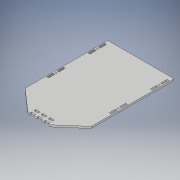
# Autodesk Inventor part: base
Saved by Autodesk Inventor 2018 (Build 220112000, 112)
## iProperties
Created: 2018-03-27
Part Number: base
Material: Generic
Document SubType Name: Modeling
Designer: guita
Density: 1 g/cm^3
Appearance: Default
Author: guita
Autodesk Inventor part; units mm, degrees
ref_plane "YZ Plane" through (0, 0, 0) normal (1, 0, 0) x (0, 1, 0)
ref_plane "XZ Plane" through (0, 0, 0) normal (0, 1, 0) x (-1, 0, 0)
ref_plane "XY Plane" through (0, 0, 0) normal (0, 0, 1) x (1, 0, 0)
sketch "Sketch1" plane through (0, 0, 0) normal (0, 1, 0) x (-1, 0, 0)
  point P0 (0, 0)
sketch "Sketch4" plane through (0, 0, 0) normal (0, 1, 0) x (-1, 0, 0)
  line L0 (-203.2, 0) -> (-203.2, -254)
  line L1 (-203.2, -254) -> (0, -254)
  line L2 (0, -254) -> (0, 0)
  line L3 (-101.6, 44.45) -> (-50.8, 44.45)
  line L4 (-50.8, 44.45) -> (0, 0)
  line L5 (-101.6, 44.45) -> (-152.4, 44.45)
  line L6 (-152.4, 44.45) -> (-203.2, 0)
  line L7 (-152.4, 44.45) -> (-136.0714, 58.7375)
  line L8 (-50.8, 44.45) -> (-67.1286, 58.7375)
  line L9 (-67.1286, 58.7375) -> (-136.0714, 58.7375)
  line L10 (0, -254) -> (0, -241.3)
  line L11 (-3.175, -241.3) -> (-3.175, -222.25)
  line L12 (-3.175, -222.25) -> (-9.525, -222.25)
  line L13 (-9.525, -222.25) -> (-9.525, -241.3)
  line L14 (-9.525, -241.3) -> (-3.175, -241.3)
  circle A0 centre (-6.35, -215.9) radius 4.7625
  circle A1 centre (-6.35, -215.9) radius 1.9844
  line L15 (-6.35, -209.55) -> (-9.525, -209.55)
  line L16 (-6.35, -209.55) -> (-3.175, -209.55)
  line L17 (-3.175, -209.55) -> (-3.175, -190.5)
  line L18 (-3.175, -190.5) -> (-9.525, -190.5)
  line L19 (-9.525, -190.5) -> (-9.525, -209.55)
  line L20 (-200.025, -241.3) -> (-200.025, -222.25)
  line L21 (-200.025, -222.25) -> (-193.675, -222.25)
  line L22 (-193.675, -222.25) -> (-193.675, -241.3)
  line L23 (-193.675, -241.3) -> (-200.025, -241.3)
  circle A2 centre (-196.85, -215.9) radius 4.7625
  circle A3 centre (-196.85, -215.9) radius 1.9844
  line L24 (-196.85, -209.55) -> (-193.675, -209.55)
  line L25 (-196.85, -209.55) -> (-200.025, -209.55)
  line L26 (-200.025, -209.55) -> (-200.025, -190.5)
  line L27 (-200.025, -190.5) -> (-193.675, -190.5)
  line L28 (-193.675, -190.5) -> (-193.675, -209.55)
  line L29 (-3.175, -63.5) -> (-3.175, -82.55)
  line L30 (-3.175, -82.55) -> (-9.525, -82.55)
  line L31 (-9.525, -82.55) -> (-9.525, -63.5)
  line L32 (-9.525, -63.5) -> (-3.175, -63.5)
  circle A4 centre (-6.35, -88.9) radius 4.7625
  circle A5 centre (-6.35, -88.9) radius 1.9844
  line L33 (-6.35, -95.25) -> (-9.525, -95.25)
  line L34 (-6.35, -95.25) -> (-3.175, -95.25)
  line L35 (-3.175, -95.25) -> (-3.175, -114.3)
  line L36 (-3.175, -114.3) -> (-9.525, -114.3)
  line L37 (-9.525, -114.3) -> (-9.525, -95.25)
  line L38 (-193.675, -63.5) -> (-200.025, -63.5)
  line L39 (-200.025, -63.5) -> (-200.025, -82.55)
  line L40 (-193.675, -82.55) -> (-193.675, -63.5)
  line L41 (-200.025, -82.55) -> (-193.675, -82.55)
  circle A6 centre (-196.85, -88.9) radius 4.7625
  line L42 (-196.85, -95.25) -> (-200.025, -95.25)
  line L43 (-196.85, -95.25) -> (-193.675, -95.25)
  line L44 (-200.025, -95.25) -> (-200.025, -114.3)
  line L45 (-200.025, -114.3) -> (-193.675, -114.3)
  line L46 (-193.675, -114.3) -> (-193.675, -95.25)
  circle A7 centre (-196.85, -88.9) radius 1.9844
  dimension "d18" = 203.2
  dimension "d19" = 254
  dimension "d29" = 19.05
  dimension "d30" = 6.35
  dimension "d32" = 9.525
  dimension "d33" = 3.9688
  dimension "d35" = 3.175
  dimension "d36" = 19.05
  constraints: 94 end point, 8 centre point, 6 perpendicular, 5 horizontal, 4 coincident, 2 parallel, 2 point on line
  measures "d18" distance of L1.end L0.end
  measures "d19" distance of L0.end L0.start
  measures "d29" distance of L11.start L11.end
  measures "d30" distance of L11.end L12.end
  measures "d32" diameter of A0
  measures "d33" diameter of A1
  measures "d35" distance of L15.start L16.end
  measures "d36" distance of L16.end L17.end
extrude "Extrusion2" add sketch "Sketch4" along normal blind 5.5563 contours L6 L5 L3 L4 L2 L1 L0 | L7 L9 L8 L3 L5 | A0 | A2 | A4 | A6
sketch "Sketch5" plane through (0, 5.5563, 0) normal (0, 1, 0) x (1, 0, 0)
  line L0 (67.1286, -58.7375) -> (136.0714, -58.7375) projected
  line L1 (136.0714, -58.7375) -> (129.7214, -58.7375)
  line L2 (129.7214, -58.7375) -> (129.7214, -52.3875)
  line L3 (129.7214, -52.3875) -> (117.0214, -52.3875)
  line L4 (117.0214, -52.3875) -> (117.0214, -58.7375)
  line L5 (117.0214, -58.7375) -> (104.3214, -58.7375)
  line L6 (0, 0) -> (67.1286, -58.7375) projected
  line L7 (67.1286, -58.7375) -> (73.4786, -58.7375)
  line L8 (73.4786, -58.7375) -> (73.4786, -52.3875)
  line L9 (73.4786, -52.3875) -> (86.1786, -52.3875)
  line L10 (86.1786, -52.3875) -> (86.1786, -58.7375)
  line L11 (86.1786, -58.7375) -> (101.5964, -58.7375)
  line L12 (101.5964, -52.3875) -> (95.2464, -52.3875)
  line L13 (101.5964, -52.3875) -> (107.9464, -52.3875)
  line L14 (107.9464, -52.3875) -> (107.9464, -58.7375)
  line L15 (95.2464, -52.3875) -> (95.2464, -58.7375)
  line L16 (73.4786, -58.7375) -> (86.1786, -58.7375)
  constraints: 30 end point, 8 perpendicular, 7 point on line, 1 collinear, 1 horizontal
extrude "Extrusion3" cut sketch "Sketch5" against normal blind 25.4
sketch "Sketch6" plane through (0, 5.5563, 0) normal (0, 1, 0) x (1, 0, 0)
  line L0 (73.4786, -52.3875) -> (86.1786, -52.3875) projected
  line L1 (73.4786, -46.0375) -> (73.4786, -39.6875)
  line L2 (73.4786, -39.6875) -> (73.4786, -46.0375)
  line L3 (129.74, -46.0375) -> (129.74, -39.6875)
  line L4 (129.74, -39.6875) -> (129.74, -46.0375)
  line L5 (86.1786, -46.0375) -> (86.1786, -39.6875)
  line L6 (95.2464, -46.0375) -> (95.2464, -39.6875)
  line L7 (117.0167, -46.0375) -> (117.0167, -39.6875)
  line L8 (107.95, -46.0375) -> (107.95, -39.6875)
  line L9 (73.4786, -39.6875) -> (86.1786, -39.6875)
  line L10 (95.2464, -39.6875) -> (107.95, -39.6875)
  line L11 (117.0167, -39.6875) -> (129.74, -39.6875)
  line L12 (129.74, -46.0375) -> (117.0167, -46.0375)
  line L13 (107.95, -46.0375) -> (95.2464, -46.0375)
  line L14 (86.1786, -46.0375) -> (73.4786, -46.0375)
  point P0 (0, 0)
  point P1 (95.2464, -52.3875)
  constraints: 28 end point, 15 perpendicular, 2 vertical
extrude "Extrusion4" cut sketch "Sketch6" against normal blind 25.4
sketch "Sketch7" plane through (0, 5.5563, 0) normal (0, 1, 0) x (1, 0, 0)
  line L0 (3.175, 63.5) -> (3.175, 82.55) projected
  line L1 (3.175, 73.025) -> (8.7313, 73.025)
  line L2 (9.525, 82.55) -> (3.175, 82.55) projected
  line L3 (3.175, 63.5) -> (9.525, 63.5) projected
  line L4 (9.525, 82.55) -> (8.7313, 82.55)
  line L5 (8.7313, 82.55) -> (8.7313, 63.5)
  line L6 (8.7313, 63.5) -> (9.525, 63.5)
  line L7 (9.525, 63.5) -> (9.525, 82.55)
  line L8 (9.525, 114.3) -> (8.7313, 114.3)
  line L9 (8.7313, 114.3) -> (8.7313, 95.25)
  line L10 (8.7313, 95.25) -> (9.525, 95.25)
  line L11 (9.525, 95.25) -> (9.525, 114.3)
  line L12 (3.175, 209.55) -> (9.525, 209.55) projected
  line L13 (3.175, 190.5) -> (9.525, 190.5) projected
  line L14 (9.525, 209.55) -> (8.7313, 209.55)
  line L15 (8.7313, 209.55) -> (8.7313, 190.5)
  line L16 (8.7313, 190.5) -> (9.525, 190.5)
  line L17 (9.525, 190.5) -> (9.525, 209.55)
  line L18 (9.525, 241.3) -> (9.525, 222.25) projected
  line L19 (9.525, 241.3) -> (9.1281, 241.3)
  line L20 (9.1281, 222.25) -> (9.525, 222.25)
  line L21 (9.525, 222.25) -> (9.525, 241.3)
  line L22 (3.175, 222.25) -> (3.175, 241.3) projected
  line L23 (9.525, 241.3) -> (8.7313, 241.3)
  line L24 (8.7313, 241.3) -> (8.7313, 222.25)
  line L25 (8.7313, 222.25) -> (9.525, 222.25)
  line L26 (9.525, 222.25) -> (9.525, 241.3)
  line L27 (200.025, 241.3) -> (200.025, 222.25) projected
  line L28 (200.025, 231.775) -> (194.4688, 231.775)
  line L29 (193.675, 241.3) -> (193.675, 222.25) projected
  line L30 (193.675, 241.3) -> (194.4688, 241.3)
  line L31 (194.4688, 241.3) -> (194.4688, 222.25)
  line L32 (194.4688, 222.25) -> (193.675, 222.25)
  line L33 (193.675, 222.25) -> (193.675, 241.3)
  line L34 (193.675, 209.55) -> (193.675, 190.5) projected
  line L35 (200.025, 190.5) -> (193.675, 190.5) projected
  line L36 (193.675, 209.55) -> (194.4688, 209.55)
  line L37 (194.4688, 209.55) -> (194.4688, 190.5)
  line L38 (194.4688, 190.5) -> (193.675, 190.5)
  line L39 (193.675, 190.5) -> (193.675, 209.55)
  line L40 (193.675, 114.3) -> (194.4688, 114.3)
  line L41 (194.4688, 114.3) -> (194.4688, 95.25)
  line L42 (194.4688, 95.25) -> (193.675, 95.25)
  line L43 (193.675, 95.25) -> (193.675, 114.3)
  line L44 (193.675, 82.55) -> (193.675, 63.5) projected
  line L45 (193.675, 82.55) -> (194.4688, 82.55)
  line L46 (194.4688, 82.55) -> (194.4688, 63.5)
  line L47 (194.4688, 63.5) -> (193.675, 63.5)
  line L48 (193.675, 63.5) -> (193.675, 82.55)
  line L49 (86.1786, -52.3875) -> (86.1786, -58.7375) projected
  line L50 (73.4786, -52.3875) -> (73.4786, -58.7375) projected
  line L51 (86.1786, -52.3875) -> (73.4786, -52.3875)
  line L52 (73.4786, -52.3875) -> (73.4786, -53.1813)
  line L53 (73.4786, -53.1813) -> (86.1786, -53.1813)
  line L54 (86.1786, -53.1813) -> (86.1786, -52.3875)
  line L55 (95.2464, -58.7375) -> (95.2464, -52.3875) projected
  line L56 (107.9464, -52.3875) -> (107.9464, -58.7375) projected
  line L57 (95.2464, -52.3875) -> (107.9464, -52.3875)
  line L58 (107.9464, -52.3875) -> (107.9464, -53.1813)
  line L59 (107.9464, -53.1813) -> (95.2464, -53.1813)
  line L60 (95.2464, -53.1813) -> (95.2464, -52.3875)
  line L61 (117.0214, -52.3875) -> (130.175, -52.3875)
  line L62 (130.175, -52.3875) -> (130.175, -53.1813)
  line L63 (130.175, -53.1813) -> (117.0214, -53.1813)
  line L64 (117.0214, -53.1813) -> (117.0214, -52.3875)
  line L65 (86.1786, -46.0375) -> (86.1786, -39.6875) projected
  line L66 (73.4786, -39.6875) -> (86.1786, -39.6875)
  line L67 (86.1786, -39.6875) -> (86.1786, -40.4853)
  line L68 (86.1786, -40.4853) -> (73.4786, -40.4853)
  line L69 (73.4786, -40.4853) -> (73.4786, -39.6875)
  line L70 (95.2464, -39.6875) -> (107.9464, -39.6875)
  line L71 (107.9464, -39.6875) -> (107.9464, -40.4853)
  line L72 (107.9464, -40.4853) -> (95.2464, -40.4853)
  line L73 (95.2464, -40.4853) -> (95.2464, -39.6875)
  line L74 (117.0214, -39.6875) -> (129.74, -39.6875)
  line L75 (129.74, -39.6875) -> (129.74, -40.4853)
  line L76 (129.74, -40.4853) -> (117.0214, -40.4853)
  line L77 (117.0214, -40.4853) -> (117.0214, -39.6875)
  point P0 (0, 0)
  dimension "d65" = 5.5563
  dimension "d67" = 5.5563
  constraints: 122 end point, 29 parallel, 18 point on line, 17 horizontal, 14 perpendicular, 2 midpoint
  measures "d65" distance of L1.start L1.end
  measures "d67" distance of L28.start L28.end
extrude "Extrusion5" add sketch "Sketch7" against normal blind 5.5563 contours L5 L2 L7 L3 | L11 L10 L9 L8 | L12 L17 L13 L15 | L18 L20 L25 L24 L23 L19 | L30 L31 L32 L29 | L36 L37 L35 L34 | L40 L41 L42 L43 | L45 L46 L47 L44 | L49 L53 L50 L51 | L55 L57 L56 L59 | L61 L62 L63 L64 | L68 L69 L66 L65 | L70 L71 L72 L73 | L74 L75 L76 L77
body "Solid2"
